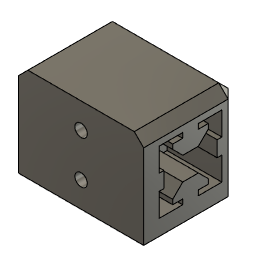
Interchange (Autodesk Fusion 360 design; units mm, degrees)
Autodesk Fusion 360 part; units mm, degrees
note: some values were not read from the file. Set by a fixed rule: which sketch regions a step uses.
sketch "Sketch1" plane through (0, 0, 0) normal (1, 0, 0) x (0, 0, -1)
  line L0 (0, 0) -> (5, 0)
  line L1 (5, 0) -> (5, -5)
  line L2 (5, -5) -> (-25, -5)
  line L3 (-25, -5) -> (-25, 25)
  line L4 (-25, 25) -> (5, 25)
  line L5 (5, 25) -> (5, -5)
  line L6 (0, 0) -> (-20, 0)
  line L7 (-20, 0) -> (-20, 20)
  line L8 (-20, 20) -> (0, 20)
  line L9 (0, 20) -> (0, 0)
  line L10 (-12.5, 20) -> (-7.5, 20)
  line L11 (-7.5, 20) -> (-7.5, 13.7)
  line L12 (-7.5, 13.7) -> (-12.5, 13.7)
  line L13 (-12.5, 13.7) -> (-12.5, 20)
  line L14 (-12.5, 0) -> (-7.5, 0)
  line L15 (-7.5, 0) -> (-7.5, 6.3)
  line L16 (-7.5, 6.3) -> (-12.5, 6.3)
  line L17 (-12.5, 6.3) -> (-12.5, 0)
  line L18 (-18.5, 7.5) -> (-20, 7.5)
  line L19 (-20, 7.5) -> (-20, 12.5)
  line L20 (-20, 12.5) -> (-18.5, 12.5)
  line L21 (-18.5, 12.5) -> (-18.5, 7.5)
  line L22 (-1.5, 7.5) -> (0, 7.5)
  line L23 (0, 7.5) -> (0, 12.5)
  line L24 (0, 12.5) -> (-1.5, 12.5)
  line L25 (-1.5, 12.5) -> (-1.5, 7.5)
  constraint coincident L0.start L6.start
  constraint horizontal L0
  constraint perpendicular L0 L1
  constraint horizontal L2
  constraint vertical L3
  constraint horizontal L4
  constraint vertical L5
  constraint horizontal L6
  constraint vertical L7
  constraint horizontal L8
  constraint vertical L9
  constraint horizontal L10
  constraint vertical L11
  constraint horizontal L12
  constraint vertical L13
  constraint coincident L8 L10.start
  constraint horizontal L14
  constraint vertical L15
  constraint horizontal L16
  constraint vertical L17
  constraint coincident L6 L14.start
  constraint horizontal L18
  constraint vertical L19
  constraint horizontal L20
  constraint vertical L21
  constraint horizontal L22
  constraint vertical L23
  constraint horizontal L24
  constraint vertical L25
  constraint coincident L9 L23.end
extrude "Extrude1" add sketch "Sketch1" along normal blind 70 contours L1 L2 L3 L4 L5 | L6 L14 L15 L16 L17 | L9 L22 L23 L24 L25 | L7 L18 L19 L20 L21 | L8 L10 L11 L12 L13
sketch "Sketch2" plane through (0, 0, 0) normal (1, 0, 0) x (0, 0, -1)
  line L0 (-12.5, 13.7) -> (-20, 13.7)
  line L1 (-20, 13.7) -> (-20, 20)
  line L2 (-20, 20) -> (-12.5, 20)
  line L3 (-12.5, 20) -> (-12.5, 13.7)
  line L4 (-7.5, 13.7) -> (0, 13.7)
  line L5 (0, 13.7) -> (0, 20)
  line L6 (0, 20) -> (-7.5, 20)
  line L7 (-7.5, 20) -> (-7.5, 13.7)
  line L8 (-7.5, 6.3) -> (0, 6.3)
  line L9 (0, 6.3) -> (0, 0)
  line L10 (0, 0) -> (-7.5, 0)
  line L11 (-7.5, 0) -> (-7.5, 6.3)
  line L12 (-12.5, 6.3) -> (-20, 6.3)
  line L13 (-20, 6.3) -> (-20, 0)
  line L14 (-20, 0) -> (-12.5, 0)
  line L15 (-12.5, 0) -> (-12.5, 6.3)
  constraint horizontal L0
  constraint vertical L1
  constraint horizontal L2
  constraint vertical L3
  constraint horizontal L4
  constraint vertical L5
  constraint horizontal L6
  constraint vertical L7
  constraint horizontal L8
  constraint vertical L9
  constraint horizontal L10
  constraint vertical L11
  constraint coincident L9.end L10.start
  constraint horizontal L12
  constraint vertical L13
  constraint horizontal L14
  constraint vertical L15
extrude "Extrude2" add sketch "Sketch2" along normal blind 30 and the other way blind -40
extrude "Extrude3" cut 4 faces at (40, 15.8, 15) (40, 15.8, 5) (40, 4.2, 5) (40, 4.2, 17.5) along direction (-1, 0, 0) blind 2.5
extrude "Extrude4" cut 4 faces at (30, 15.8, 5) (30, 15.8, 15) (30, 4.2, 5) (30, 4.2, 17.5) along direction (1, 0, 0) blind 2.5
extrude "Extrude5" cut 1 faces at (0, 10.8333, 23.3333) along direction (1, 0, 0) blind 15
extrude "Extrude6" cut 1 faces at (70, 10.8333, 23.3333) along direction (-1, 0, 0) blind 15
sketch "Sketch3" plane through (0, 0, 0) normal (1, 0, 0) x (0, 0, -1)
  line L0 (-12.5, 6.3) -> (-15.7, 3.1)
  line L1 (-15.7, 3.1) -> (-15.7, 1.6)
  line L2 (-15.7, 1.6) -> (-12.5, 1.6)
  line L3 (-7.5, 6.3) -> (-4.3, 3.1)
  line L4 (-4.3, 3.1) -> (-4.3, 1.6)
  line L5 (-4.3, 1.6) -> (-12.5, 1.6)
  line L6 (-12.5, 6.3) -> (-7.5, 6.3)
  line L7 (-7.5, 13.7) -> (-4.3, 16.9)
  line L8 (-4.3, 16.9) -> (-4.3, 18.4)
  line L9 (-4.3, 18.4) -> (-15.7, 18.4)
  line L10 (-15.7, 18.4) -> (-15.7, 16.9)
  line L11 (-15.7, 16.9) -> (-12.5, 13.7)
  line L12 (-12.5, 13.7) -> (-7.5, 13.7)
  constraint vertical L1
  constraint perpendicular L1 L2
  constraint perpendicular L0 L3
  constraint perpendicular L2 L4
  constraint perpendicular L4 L5
  constraint parallel L5 L6
  constraint perpendicular L3 L7
  constraint perpendicular L6 L8
  constraint perpendicular L1 L9
  constraint perpendicular L9 L10
  constraint perpendicular L0 L11
  constraint parallel L9 L12
extrude "Extrude7" add sketch "Sketch3" along normal blind 55 and the other way blind -15
chamfer "Chamfer1" distance 3 angle 45 5 edges at (15, 25, 10) (55, 25, 10) (35, 25, -5) (55, 10, -5) (15, 10, -5)
sketch "Sketch4" plane through (0, 0, 25) normal (0, 0, 1) x (1, 0, 0)
  line L0 (55, 22) -> (52, 25)
  line L1 (52, 25) -> (18, 25)
  line L2 (18, 25) -> (15, 22)
  line L3 (15, 22) -> (15, -5)
  line L4 (15, -5) -> (55, -5)
  line L5 (55, -5) -> (55, 22)
  line L6 (35, 10) -> (35, 3.15)
  line L7 (35, 10) -> (35, 16.85)
  circle A0 centre (35, 16.85) radius 2
  circle A1 centre (35, 3.15) radius 2
  dimension "d20" = 6.85
  dimension "d21" = 6.85
  dimension "d22" = 4
  dimension "d23" = 4
  constraint perpendicular L1 L6
  constraint parallel L6 L7
  constraint coincident L7.end A0.centre
  constraint coincident L6.end A1.centre
  measures "d20" distance of L6.start L6.end
  measures "d21" distance of L6.start L7.end
  measures "d22" diameter of A0
  measures "d23" diameter of A1
extrude "Extrude8" cut sketch "Sketch4" against normal blind 30 contours A0 | A1
